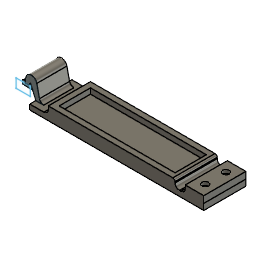
krishka_sanyo_otgninaysha (Autodesk Fusion 360 design; units mm, degrees)
Autodesk Fusion 360 part; units mm, degrees
sketch "Sketch1" plane through (0, 0, 0) normal (0, 1, 0) x (1, 0, 0)
  line L0 (32.5, 9.65) -> (-32.5, 9.65)
  line L1 (-32.5, 9.65) -> (-32.5, -9.65)
  line L2 (-32.5, -9.65) -> (32.5, -9.65)
  line L3 (32.5, -9.65) -> (32.5, 9.65)
  line L4 (32.5, 9.65) -> (-32.5, -9.65) construction
  line L5 (-32.5, 9.65) -> (32.5, -9.65) construction
  line L6 (32.5, 9.65) -> (34.5, 9.65)
  line L7 (34.5, 9.65) -> (34.5, -9.35)
  line L8 (34.5, -9.35) -> (32.5, -9.35)
  line L9 (32.5, -9.35) -> (32.5, 9.65)
  line L10 (-32.5, 9.65) -> (-37.5, 9.65)
  line L11 (-37.5, 9.65) -> (-37.5, -9.5)
  line L12 (-37.5, -9.5) -> (-32.5, -9.5)
  line L13 (-32.5, -9.5) -> (-32.5, 9.65)
  dimension "d1" = 65
  dimension "d2" = 19.3
  dimension "d3" = 2
  dimension "d4" = 19
  dimension "d5" = 5
  constraint horizontal L0
  constraint perpendicular L0 L1
  constraint parallel L0 L2
  constraint parallel L1 L3
  constraint coincident L4 origin
  constraint coincident L5 origin
  constraint horizontal L6
  constraint vertical L7
  constraint horizontal L8
  constraint vertical L9
  constraint horizontal L10
  constraint vertical L11
  constraint horizontal L12
  constraint vertical L13
  measures "d1" distance of L1.end L2.end
  measures "d2" distance of L0.end L1.end
  measures "d3" distance of L0.start L6.end
  measures "d4" distance of L0.start L8.end
  measures "d5" distance of L0.end L10.end
extrude "Extrude1" add sketch "Sketch1" along normal blind 5.5 contours L0 L1 L2 L3 L9 L13
extrude "Extrude2" add sketch "Sketch1" along normal blind 2 contours L3 L6 L7 L8 L9
extrude "Extrude3" add sketch "Sketch1" along normal blind 2 contours L1 L10 L11 L12 L13
sketch "Sketch2" plane through (0, 0, 9.65) normal (0, 0, 1) x (1, 0, 0)
  line L0 (-32.5, 0) -> (32.5, 0)
  line L1 (34.5, 0) -> (34.5, 2)
  line L2 (34.5, 2) -> (32.5, 2)
  line L3 (32.5, 0) -> (32.5, 5.5)
  line L4 (32.5, 5.5) -> (-32.5, 5.5)
  line L5 (-32.5, 5.5) -> (-32.5, 0)
  line L6 (-32.5, 2) -> (-37.5, 2)
  line L7 (-37.5, 2) -> (-37.5, 0)
  line L8 (33.6424, 5.5) -> (42.1424, 5.5)
  line L9 (33.6424, 5.5) -> (33.6424, 2.4499)
  line L10 (42.1424, 5.5) -> (42.1424, 2.4499)
  line L11 (42.1424, 2.4499) -> (33.6424, 2.4499)
  line L12 (-32.5, 0) -> (-40.5, 0)
  line L13 (-45.0976, 3.4495) -> (-41.0979, 3.4562)
  line L14 (-40.5987, 3.957) -> (-40.6027, 6.3116)
  line L15 (-42.5164, 5.4956) -> (-45.1003, 5.4913)
  line L16 (-45.5995, 4.9908) -> (-45.5984, 3.949)
  line L17 (-37.5, 2) -> (-39.8153, 7.5767)
  line L18 (-40.1899, 7.5627) -> (-40.6027, 6.3116)
  arc A0 (-39.8153, 7.5767) -> (-40.1899, 7.5627) centre (-40, 7.5) ccw
  arc A1 (-45.1003, 5.4913) -> (-45.5995, 4.9908) centre (-45.0995, 4.9913) ccw
  arc A2 (-45.5984, 3.949) -> (-45.0976, 3.4495) centre (-45.0984, 3.9495) ccw
  arc A3 (-41.0979, 3.4562) -> (-40.5987, 3.957) centre (-41.0987, 3.9562) ccw
  line L19 (33.6424, 2.4499) -> (33.6424, 2)
  line L20 (-35.4489, 2) -> (-36.9951, 9.0494)
  arc A4 (-36.9951, 9.0494) -> (-42.0393, 8.86) centre (-39.5001, 8.4999) ccw
  line L21 (-42.0393, 8.86) -> (-42.5164, 5.4956)
  line L22 (32.5, 0) -> (34.5, 0)
  line L23 (32.5, 2) -> (32.5, 0)
  line L24 (-37.5, 0) -> (-32.5, 0)
  line L25 (-32.5, 0) -> (-32.5, 2)
  line L26 (34.5, 2) -> (34.5, 2.4499)
  point P0 (-45.5979, 3.4487)
  point P1 (-40.5979, 3.457)
  dimension "d12" = 8.5
  dimension "d41" = 8
  dimension "d42" = 5
  dimension "d44" = 0.2
  dimension "d45" = 0.5
  dimension "d46" = 0.5
  dimension "d47" = 0.5
  constraint perpendicular L2 L9
  constraint perpendicular L8 L10
  constraint perpendicular L9 L11
  constraint coincident L0.start L5.end
  constraint perpendicular L7 L12
  constraint perpendicular L13 L14
  constraint perpendicular L14 L15
  constraint coincident L6.end L7.start
  constraint tangent L17 A0
  constraint tangent L18 A0
  constraint tangent L15 A1
  constraint tangent L16 A1
  constraint coincident P0 L13
  constraint coincident P0 L16
  constraint tangent L13 A2
  constraint tangent L16 A2
  constraint coincident P1 L13
  constraint coincident P1 L14
  constraint tangent L13 A3
  constraint tangent L14 A3
  constraint coincident L2 L19.end
  constraint tangent L20 A4
  constraint tangent A4 L21
  constraint coincident L6 L20.start
  constraint coincident L1.end L2.start
  constraint coincident L11 L26.end
  constraint perpendicular L11 L26
  measures "d12" distance of L8.start L8.end
  measures "d41" distance of L0.start L12.end
  measures "d42" distance of P0 P1
  measures "d44" radius of A0
  measures "d45" radius of A1
  measures "d46" radius of A2
  measures "d47" radius of A3
extrude "Extrude4" add sketch "Sketch2" against normal blind 19.2 contours L1 L2 L3 L22 L23 | L2 L11 L19 L26 | L8 L9 L10 L11
extrude "Extrude5" add sketch "Sketch2" along normal blind -19.3 and the other way blind 2.5 contours L5 L6 L7 L12 L24 L25 | L1 L2 L3 L22 L23 | L2 L11 L19 L26 | L8 L9 L10 L11
fillet "Fillet1" radius 1 1 edges at (-32.5, 5.5, 0)
fillet "Fillet2" radius 1 1 edges at (32.5, 5.5, 0)
sketch "Sketch3" plane through (0, 5.5, 0) normal (0, 1, 0) x (-1, 0, 0)
  line L0 (-33.6424, 9.65) -> (-42.1424, 9.65)
  line L1 (-42.1424, 9.65) -> (-42.1424, -9.65)
  line L2 (-42.1424, -9.65) -> (-33.6424, -9.65)
  line L3 (-33.6424, -9.65) -> (-33.6424, 9.65)
  line L4 (-33.6424, 0) -> (-42.1424, 0)
  circle A0 centre (-37.8924, -4.75) radius 1.5
  circle A1 centre (-37.8924, -4.75) radius 2.5
  circle A2 centre (-37.8924, 4.75) radius 2.5
  circle A3 centre (-37.8924, 4.75) radius 1.5
  dimension "d31" = 3
  dimension "d32" = 5
  constraint midpoint L3 L4.start
  constraint midpoint L1 L4.end
  constraint concentric A0 A1
  constraint symmetric L4 A0 A3
  constraint symmetric L4 A1 A2
  measures "d31" diameter of A0
  measures "d32" diameter of A1
extrude "Extrude6" cut sketch "Sketch3" against normal blind 6 contours A0 | A3
extrude "Extrude10" add 1 faces at (34.5, 1.4833, 3.2167) along direction (1, 0, 0) blind 7.642
extrude "Extrude7" cut sketch "Sketch3" along normal blind -5.5 and the other way blind 1.5 contours A0 | A1 | A2 | A3
sketch "Sketch6" plane through (0, 5.5, 0) normal (0, 1, 0) x (-1, 0, 0)
  line L0 (-31.5, 9.65) -> (-31.5, -9.65)
  line L1 (-31.5, -9.65) -> (31.5, -9.65)
  line L2 (31.5, -9.65) -> (31.5, 9.65)
  line L3 (31.5, 9.65) -> (-31.5, 9.65)
  line L4 (31.5, 9.65) -> (-31.5, 9.65)
  line L5 (-31.5, 9.65) -> (-31.5, -9.65)
  line L6 (-31.5, -9.65) -> (31.5, -9.65)
  line L7 (31.5, -9.65) -> (31.5, 9.65)
  line L8 (-29, -7.15) -> (29, -7.15)
  line L9 (29, -9.65) -> (29, 9.65)
  line L10 (29, 7.15) -> (-29, 7.15)
  line L11 (-29, 7.15) -> (-29, -7.15)
  line L12 (-26.5, 7.15) -> (-26.5, -7.15)
  line L13 (-29, 7.15) -> (-29, 9.65)
  line L14 (-29, -7.15) -> (-29, -9.65)
  line L15 (-31.5, 9.65) -> (-32.5, 9.65)
  line L16 (-32.5, 9.65) -> (-32.5, -9.65)
  line L17 (-32.5, -9.65) -> (-31.5, -9.65)
  line L18 (31.5, -9.65) -> (32.5, -9.65)
  line L19 (32.5, -9.65) -> (32.5, 9.65)
  line L20 (32.5, 9.65) -> (31.5, 9.65)
  line L21 (31.5, 9.65) -> (31.5, -9.65)
  line L22 (26.5, -7.15) -> (26.5, 7.15)
  line L23 (29, 0) -> (29, 7.15)
  dimension "d58" = -2.5
  dimension "d69" = -2.5
  constraint horizontal L4
  constraint perpendicular L4 L5
  constraint parallel L4 L6
  constraint parallel L5 L7
  constraint coincident L2.end L3.start
  constraint coincident L4 L13.end
  constraint perpendicular L4 L13
  constraint coincident L6 L14.end
  constraint perpendicular L6 L14
  constraint coincident L0.start L3.end
  constraint perpendicular L5 L15
  constraint perpendicular L4 L16
  constraint coincident L0.end L1.start
  constraint coincident L8 L12.end
  constraint coincident L10 L12.start
  constraint horizontal L18
  constraint vertical L19
  constraint horizontal L20
  constraint vertical L21
  constraint coincident L1.end L2.start
  constraint coincident L9 L23.start
  constraint coincident L8.end L9
  constraint coincident L3 L9.end
  constraint coincident L10.start L9
  constraint coincident L1 L9.start
extrude "Extrude11" cut sketch "Sketch6" against normal blind 2.5 contours L8 L10 L12 L22
extrude "Extrude12" cut sketch "Sketch6" against normal blind 3.5 contours L0 L1 L3 L4 L5 L6 L11 L13 L14 | L0 L5 L15 L16 L17 | L1 L2 L3 L4 L6 L7 L9 L21 L23 | L2 L7 L18 L19 L20 L21
fillet "Fillet4" radius 1 1 edges at (29, 5.5, 0)
extrude "Extrude14" add sketch "Sketch2" along normal blind -16.55 and the other way blind 2.75 contours L5 L6 L7 L12 L24 L25 | L6 L13 L14 L15 L16 L17 L18 A0 A1 A2 A3 L20 A4 L21
extrude "Extrude15" add sketch "Sketch2" against normal blind 0.8 contours L5 L6 L7 L12 L24 L25
fillet "Fillet5" radius 2 2 edges at (33.6424, 2, 0) (29, 2, 0)
fillet "Fillet6" radius 2 2 edges at (-35.4489, 2, 0) (-29, 2, 0)
extrude "Extrude16" add 1 faces at (-13.1932, 0, 1.4591) along direction (0, -1, 0) blind 0.4
sketch "Sketch8" plane through (0, 0, 6.9) normal (0, 0, 1) x (1, 0, 0)
  line L0 (-37.5, 2) -> (-33.84, 2)
  arc A0 (-35.7936, 3.5715) -> (-33.84, 2) centre (-33.84, 4) ccw
  line L1 (-35.7936, 3.5715) -> (-36.9951, 9.0494)
  arc A1 (-36.9951, 9.0494) -> (-42.0393, 8.86) centre (-39.5001, 8.4999) ccw
  line L2 (-42.0393, 8.86) -> (-42.5164, 5.4956)
  line L3 (-42.5164, 5.4956) -> (-45.1003, 5.4913)
  arc A2 (-45.1003, 5.4913) -> (-45.5995, 4.9908) centre (-45.0995, 4.9913) ccw
  line L4 (-45.5995, 4.9908) -> (-45.5984, 3.949)
  arc A3 (-45.5984, 3.949) -> (-45.0976, 3.4495) centre (-45.0984, 3.9495) ccw
  line L5 (-45.0976, 3.4495) -> (-41.0979, 3.4562)
  arc A4 (-41.0979, 3.4562) -> (-40.5987, 3.957) centre (-41.0987, 3.9562) ccw
  line L6 (-40.5987, 3.957) -> (-40.6027, 6.3116)
  line L7 (-40.6027, 6.3116) -> (-40.1899, 7.5627)
  arc A5 (-39.8153, 7.5767) -> (-40.1899, 7.5627) centre (-40, 7.5) ccw
  line L8 (-39.8153, 7.5767) -> (-37.5, 2)
  line L9 (-40, 6.5) -> (-46.4842, 6.4892)
  line L10 (-46.4842, 6.4892) -> (-46.4774, 2.362)
  line L11 (-46.4774, 2.362) -> (-39.9747, 2.3728)
  line L12 (-39.9747, 2.3728) -> (-40, 6.5)
  constraint perpendicular L6 L9
  constraint perpendicular L9 L10
  constraint perpendicular L10 L11
extrude "Extrude17" cut sketch "Sketch8" against normal blind 2 contours L2 L3 A2 L4 A3 L5 A4 L6 L7 L9 L10 L11 L12 | L2 L3 A2 L4 A3 L5 A4 L6 L7 L9
extrude "Extrude18" cut sketch "Sketch8" along normal blind -13.8 and the other way blind 11.8 contours L2 L3 A2 L4 A3 L5 A4 L6 L7 L9 L10 L11 L12 | L2 L3 A2 L4 A3 L5 A4 L6 L7 L9
